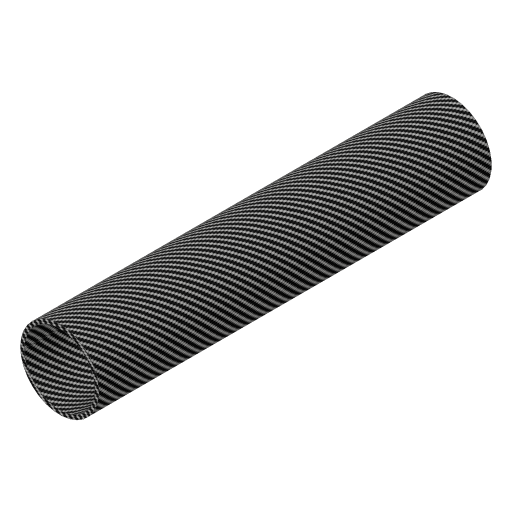
# Autodesk Inventor part: 링크2_240mm
Saved by Autodesk Inventor 2023.2 (Build 272271000, 271)
## iProperties
Created: 2021-07-06
Part Number: 링크2_240mm
Material: CFRP
Document SubType Name: Modeling
Designer: user
Density: 1.43 g/cm^3
Appearance: 탄소 섬유
Mass: 68.2857 g
Surface Area: 482.297 cm^2
Volume: 47.7522 cm^3
Author: user
Autodesk Inventor part; units mm, degrees
ref_plane "YZ Plane" through (0, 0, 0) normal (1, 0, 0) x (0, 1, 0)
ref_plane "XZ Plane" through (0, 0, 0) normal (0, 1, 0) x (-1, 0, 0)
ref_plane "XY Plane" through (0, 0, 0) normal (0, 0, 1) x (1, 0, 0)
sketch "스케치1" plane through (0, 0, 0) normal (0, 0, 1) x (1, 0, 0)
  line L0 (0, 20) -> (0, 20)
  line L1 (20, 0) -> (20, 0)
  line L2 (0, -20) -> (0, -20)
  line L3 (-20, 0) -> (-20, 0)
  line L4 (0, 18) -> (0, 18)
  line L5 (-18, 0) -> (-18, 0)
  line L6 (0, -18) -> (0, -18)
  line L7 (18, 0) -> (18, 0)
  arc A0 (0, 18) -> (-18, 0) centre (0, 0) ccw
  arc A1 (-18, 0) -> (0, -18) centre (0, 0) ccw
  arc A2 (0, -18) -> (18, 0) centre (0, 0) ccw
  arc A3 (18, 0) -> (0, 18) centre (0, 0) ccw
  arc A4 (0, 20) -> (-20, 0) centre (0, 0) ccw
  arc A5 (-20, 0) -> (0, -20) centre (0, 0) ccw
  arc A6 (0, -20) -> (20, 0) centre (0, 0) ccw
  arc A7 (20, 0) -> (0, 20) centre (0, 0) ccw
  point P0 (0, 0)
  point P1 (-20, 20)
  point P2 (20, -20)
  point P3 (20, 20)
  point P4 (-20, -20)
  point P5 (18, 18)
  point P6 (-18, 18)
  point P7 (-18, -18)
  point P8 (18, -18)
  dimension "d0" = 40
  dimension "d1" = 40
  dimension "d2" = 20
  dimension "d3" = 20
  dimension "d4" = 2
  dimension "d7" = 18
  dimension "d8" = 18
  dimension "d9" = 18
  dimension "d10" = 18
  dimension "d11" = 20
  constraints: 16 end point, 16 point on circle, 16 point on line, 16 tangent, 8 centre point, 4 parallel, 3 concentric, 2 perpendicular, 1 horizontal, 3 other
  measures "d0" distance of point (20, -20) point (-20, -20)
  measures "d1" distance of point (20, 20) point (20, -20)
  measures "d2" distance from line of L0 point (0, 0)
  measures "d3" distance from line of L3 point (0, 0)
  measures "d4" distance between parallel lines of L0 L4
  measures "d7" radius of A0
  measures "d8" radius of A1
  measures "d9" radius of A2
  measures "d10" radius of A3
  measures "d11" radius of A4
extrude "돌출1" add sketch "스케치1" along normal blind 200
equation "\"d2\" = 0.5 * d1"
equation "\"d3\" = 0.5 * d0"
